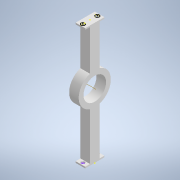
# Autodesk Inventor part: pylon
Saved by Autodesk Inventor 2021 (Build 250183000, 183)
## iProperties
Created: 2020-10-08
Part Number: pylon
Material: Generic
Document SubType Name: Modeling
Designer: bober
Density: 1 g/cm^3
Appearance: Default
Author: bober
Autodesk Inventor part; units mm, degrees
ref_plane "YZ Plane" through (0, 0, 0) normal (1, 0, 0) x (0, 1, 0)
ref_plane "XZ Plane" through (0, 0, 0) normal (0, 1, 0) x (-1, 0, 0)
ref_plane "XY Plane" through (0, 0, 0) normal (0, 0, 1) x (1, 0, 0)
sketch "Sketch4" plane through (0, 0, 0) normal (0, 1, 0) x (-1, 0, 0)
  line L0 (-10, 20) -> (10, 20)
  line L1 (10, 20) -> (10, -20)
  line L2 (10, -20) -> (-10, -20)
  line L3 (-10, -20) -> (-10, 20)
  line L4 (-10, 20) -> (10, -20) construction
  line L5 (10, 20) -> (-10, -20) construction
  point P0 (0, 0)
  dimension "d8" = 20
  dimension "d9" = 40
  constraints: 12 end point, 2 midpoint, 2 parallel, 1 horizontal, 1 perpendicular
  measures "d8" distance of L1.end L2.end
  measures "d9" distance of L0.end L1.end
extrude "Extrusion2" add sketch "Sketch4" along normal blind 3
sketch "Sketch5" plane through (0, 3, 0) normal (0, 1, 0) x (1, 0, 0)
  line L0 (10, -10) -> (-10, -10)
  line L1 (-10, -10) -> (-10, 10)
  line L2 (-10, 10) -> (10, 10)
  line L3 (10, 10) -> (10, -10)
  line L4 (10, -10) -> (-10, 10) construction
  line L5 (-10, -10) -> (10, 10) construction
  point P0 (0, 0)
  dimension "d12" = 20
  dimension "d13" = 20
  constraints: 12 end point, 2 midpoint, 2 parallel, 1 horizontal, 1 perpendicular
  measures "d12" distance of L1.end L2.end
  measures "d13" distance of L0.end L1.end
extrude "Extrusion3" add sketch "Sketch5" along normal blind 100
sketch "Sketch7" plane through (0, 3, 0) normal (0, 1, 0) x (1, 0, 0)
  circle A0 centre (0, 15) radius 2
  circle A1 centre (0, -15) radius 2
  point P0 (0, 0)
  dimension "d20" = 4
  dimension "d21" = 4
  constraints: 2 centre point
  measures "d20" diameter of A0
  measures "d21" diameter of A1
extrude "Extrusion5" cut sketch "Sketch7" against normal blind 10
sketch "Sketch8" plane through (0, 3, 0) normal (0, 1, 0) x (1, 0, 0)
  circle A0 centre (0, 15) radius 2 projected
  circle A1 centre (0, 15) radius 3.55
  circle A2 centre (0, -15) radius 2 projected
  circle A3 centre (0, -15) radius 3.55
  line L0 (2.0496, -11.45) -> (4.0992, -15)
  line L1 (4.0992, -15) -> (2.0496, -18.55)
  line L2 (2.0496, -18.55) -> (-2.0496, -18.55)
  line L3 (-2.0496, -18.55) -> (-4.0992, -15)
  line L4 (-4.0992, -15) -> (-2.0496, -11.45)
  line L5 (-2.0496, -11.45) -> (2.0496, -11.45)
  line L6 (2.0496, 18.55) -> (4.0992, 15)
  line L7 (4.0992, 15) -> (2.0496, 11.45)
  line L8 (2.0496, 11.45) -> (-2.0496, 11.45)
  line L9 (-2.0496, 11.45) -> (-4.0992, 15)
  line L10 (-4.0992, 15) -> (-2.0496, 18.55)
  line L11 (-2.0496, 18.55) -> (2.0496, 18.55)
  point P0 (0, 0)
  point P1 (0, -11.45)
  point P2 (0, 18.55)
  dimension "d24" = 7.1
  dimension "d25" = 7.1
  constraints: 24 end point, 4 coincident, 2 midpoint, 2 vertical alignment, 30 other
extrude "Extrusion6" cut sketch "Sketch8" against normal blind 3 contours A0 | A1 | A1 L6 L7 | A1 L11 L6 | L7 L8 A1 | A1 L10 L11 | L8 L9 A1 | A1 L9 L10 | A2 | A3 | A3 L0 L1 | A3 L5 L0 | L1 L2 A3 | A3 L4 L5 | L2 L3 A3 | A3 L3 L4
sketch "Sketch9" plane through (0, 0, 0) normal (0, -1, 0) x (1, 0, 0)
  line L0 (2.0496, 11.45) -> (4.0992, 15) projected
  circle A0 centre (0, 15) radius 4.0992
  circle A1 centre (0, -15) radius 4.0992
  point P0 (0, 0)
  point P1 (4.0992, -15)
  constraints: 1 horizontal alignment, 5 other
sketch "Sketch11" plane through (-10, 0, -20) normal (-1, 0, 0) x (0, 0, 1)
  line L0 (10, 0) -> (30, 0)
  line L1 (30, 0) -> (30, 250)
  line L2 (30, 250) -> (10, 250)
  line L3 (10, 250) -> (10, 0)
  arc A0 (29.9121, 100) -> (10.0879, 100) centre (20, 132) ccw projected
  line L4 (10, 250) -> (30, 250)
  line L5 (30, 250) -> (30, 163.9726)
  line L6 (30, 163.9726) -> (10, 163.9726)
  line L7 (10, 163.9726) -> (10, 250)
  point P0 (20, 0)
  point P1 (10, 163.9726)
  dimension "d29" = 250
  constraints: 16 end point, 4 parallel, 2 horizontal, 2 perpendicular, 1 point on circle, 1 point on line
  measures "d29" distance of L1.end L0.end
extrude "Extrusion7" add sketch "Sketch11" against normal blind 20 contours L3 L2 L1 A0
sketch "Sketch14" plane through (-10, 250, 10) normal (0, 1, 0) x (1, 0, 0)
  line L0 (0, 0) -> (0, -10) projected
  line L1 (20, -10) -> (20, 30) projected
  line L2 (0, -10) -> (20, -10)
  line L3 (20, -10) -> (20, 30)
  line L4 (20, 30) -> (0, 30)
  line L5 (0, 30) -> (0, -10)
  point P0 (10, 10)
  constraints: 8 end point, 2 parallel, 1 horizontal, 1 perpendicular
extrude "Extrusion8" add sketch "Sketch14" along normal blind 3
sketch "Sketch15" plane through (-10, 253, 10) normal (0, 1, 0) x (1, 0, 0)
  circle A0 centre (10, 25) radius 3.5
  circle A1 centre (10, -5) radius 3.5
  line L0 (12.0207, 28.5) -> (14.0415, 25)
  line L1 (14.0415, 25) -> (12.0207, 21.5)
  line L2 (12.0207, 21.5) -> (7.9793, 21.5)
  line L3 (7.9793, 21.5) -> (5.9585, 25)
  line L4 (5.9585, 25) -> (7.9793, 28.5)
  line L5 (7.9793, 28.5) -> (12.0207, 28.5)
  line L6 (12.0207, -1.5) -> (14.0415, -5)
  line L7 (14.0415, -5) -> (12.0207, -8.5)
  line L8 (12.0207, -8.5) -> (7.9793, -8.5)
  line L9 (7.9793, -8.5) -> (5.9585, -5)
  line L10 (5.9585, -5) -> (7.9793, -1.5)
  line L11 (7.9793, -1.5) -> (12.0207, -1.5)
  point P0 (10, 10)
  point P1 (10, 28.5)
  point P2 (10, -1.5)
  dimension "d34" = 7
  dimension "d35" = 7
  constraints: 24 end point, 4 coincident, 2 midpoint, 2 vertical alignment, 30 other
extrude "Extrusion9" cut sketch "Sketch15" against normal blind 3
sketch "Sketch16" plane through (-10, 253, 10) normal (0, 1, 0) x (1, 0, 0)
  line L0 (12.0207, 21.5) -> (14.0415, 25) projected
  circle A0 centre (10, 25) radius 4.0415
  line L1 (7.9793, -1.5) -> (12.0207, -1.5) projected
  circle A1 centre (10, -5) radius 4.0415
  point P0 (10, 10)
  constraints: 2 coincident, 6 other
sketch "Sketch17" plane through (10, 0, 20) normal (1, 0, 0) x (0, 0, -1)
  circle A0 centre (20, 133.9) radius 23.5
  circle A1 centre (20, 133.9) radius 33.5
  point P0 (20, 0)
  dimension "d38" = 47
  dimension "d39" = 67
  constraints: 2 centre point, 1 coincident
  measures "d38" diameter of A0
  measures "d39" diameter of A1
extrude "Extrusion10" add sketch "Sketch17" against normal blind 20
sketch "Sketch18" plane through (10, 0, 20) normal (1, 0, 0) x (0, 0, -1)
  point P0 (20, 0)
body "Solid2"
